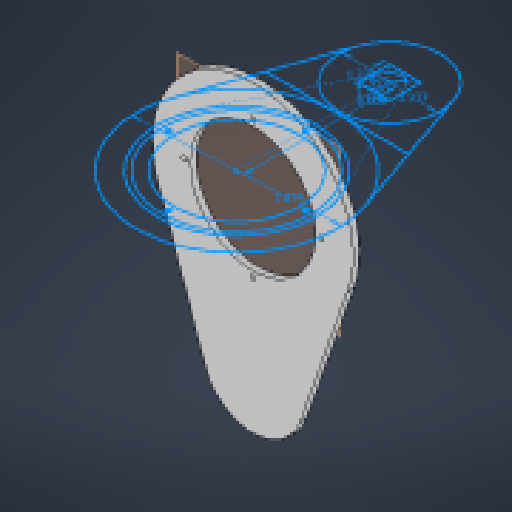
# Autodesk Inventor part: Board
Saved by Autodesk Inventor 2024 (Build 280153000, 153)
## iProperties
Created: 2023-10-21
Part Number: Board
Material: Generic
Document SubType Name: Modeling
Designer: range
Density: 1 g/cm^3
Appearance: Default
Author: range
Autodesk Inventor part; units mm, degrees
ref_plane "YZ Plane" through (0, 0, 0) normal (1, 0, 0) x (0, 1, 0)
ref_plane "XZ Plane" through (0, 0, 0) normal (0, 1, 0) x (-1, 0, 0)
ref_plane "XY Plane" through (0, 0, 0) normal (0, 0, 1) x (1, 0, 0)
ref_plane "Work Plane1" through (0, 0, 0) normal (0, 0, 1) x (1, 0, 0)
sketch "Sketch1" plane through (0, 0, 0) normal (0, 0, 1) x (1, 0, 0)
  circle A0 centre (0, -68.3) radius 2.5 projected
  circle A1 centre (-68.3, 0) radius 2.5 projected
  circle A2 centre (0, 68.3) radius 2.5 projected
  circle A3 centre (68.3, 0) radius 2.5 projected
  circle A4 centre (0, 0) radius 74.3 projected
  circle A5 centre (0, 0) radius 62.3 projected
  arc A6 (-10.8532, -157.7212) -> (10.8532, -157.7212) centre (0, -152.4) ccw construction
  circle A7 centre (0, 0) radius 79.1775 projected
  line L0 (-10.8532, -157.7212) -> (-71.0925, -34.8557) construction
  line L1 (10.8532, -157.7212) -> (71.0925, -34.8557) construction
  arc A8 (-10.8532, -157.7212) -> (10.8532, -157.7212) centre (0, -152.4) ccw
  arc A9 (71.0925, -34.8557) -> (-71.0925, -34.8557) centre (0, 0) ccw
  line L2 (0, -152.4) -> (0, 0) construction
  circle A10 centre (0, 0) radius 100
  circle A11 centre (0, -152.4) radius 50
  line L3 (-47.2324, -168.8042) -> (-94.4649, -32.8084)
  line L4 (47.2324, -168.8042) -> (94.4649, -32.8084)
  line L5 (71.1287, -100) -> (-71.1287, -100)
  line L6 (15.494, -167.894) -> (-15.494, -167.894)
  line L7 (-15.494, -167.894) -> (-15.494, -136.906)
  line L8 (-15.494, -136.906) -> (15.494, -136.906)
  line L9 (15.494, -136.906) -> (15.494, -167.894)
  line L10 (15.494, -167.894) -> (-15.494, -136.906) construction
  line L11 (-15.494, -167.894) -> (15.494, -136.906) construction
  dimension "d0" = 24.175
  dimension "d1" = 152.4
  dimension "d4" = 200
  dimension "d5" = 100
  dimension "d6" = 30.988
  dimension "d7" = 30.988
  constraints: 24 end point, 12 point on circle, 9 tangent, 5 centre point, 4 coincident, 2 horizontal, 2 midpoint, 2 parallel, 2 point on line, 1 perpendicular, 1 vertical
  measures "d0" diameter of A6
  measures "d1" distance of L2.start L2.end
  measures "d4" diameter of A10
  measures "d5" diameter of A11
  measures "d6" distance of L7.end L8.end
  measures "d7" distance of L8.end L6.start
extrude "Extrusion1" add sketch "Sketch1" along normal blind 6.35 contours A4 | A7 | A10 | A10 L5 L3 | L4 L5 A10 | L5 L4 A11 L3 | A11 | L6 L7 L8 L9
hole "Hole1" at (15.494, -136.906, 0) at (15.494, -167.894, 0) at (-15.494, -167.894, 0) at (-15.494, -136.906, 0) direction (0, 0, 1) diameter 3.4036 end through all clearance for "Flat Head Machine Screw" size "M3" standard "Ansi Metric M Profile"
body "Solid1"
